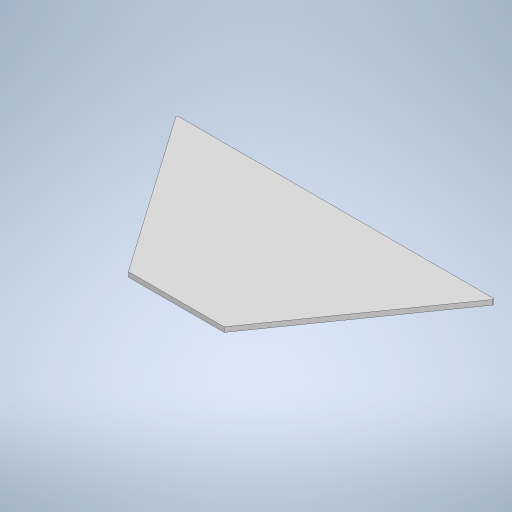
# Autodesk Inventor part: ДМС 304 торец лотка кормовой
Saved by Autodesk Inventor 2024.2 (Build 282272000, 272)
## iProperties
Created: 2024-05-13
Part Number: ДМС 304 торец лотка кормовой
Material: Generic
Document SubType Name: Sheet Metal
Designer: admin
Density: 1 g/cm^3
Sheet Metal Rule: Default
Appearance: Default
Author: admin
Autodesk Inventor part; units mm, degrees
ref_plane "YZ Plane" through (0, 0, 0) normal (1, 0, 0) x (0, 1, 0)
ref_plane "XZ Plane" through (0, 0, 0) normal (0, 1, 0) x (-1, 0, 0)
ref_plane "XY Plane" through (0, 0, 0) normal (0, 0, 1) x (1, 0, 0)
sketch "Sketch1" plane through (0, 0, 0) normal (0, 0, 1) x (1, 0, 0)
  line L0 (-100.0208, 100) -> (-30, 0)
  line L1 (-30, 0) -> (30, 0)
  line L2 (30, 0) -> (100.0208, 100)
  line L3 (100.0208, 100) -> (-100.0208, 100)
  point P0 (0, 0)
  point P1 (0, 0)
  point P2 (0, 100)
  dimension "d0" = 100
  dimension "d1" = 60
  dimension "d2" = 200.0415
  dimension "d4" = 125
  measures "d0" distance between parallel lines of L1 L3
  measures "d1" distance of L0.end L1.end
  measures "d2" distance of L2.end L0.start
  measures "d4" angle of L1 L0
extrude "Plate1" add sketch "Sketch1" along normal blind 3
chamfer "Chamfer1" distance 1 angle 45 2 edges at (-100.0208, 100, 1.5) (100.0208, 100, 1.5)
equation "\"d0\" = Лоток_высота"
equation "\"d1\" = Лоток_ширина_низ"
equation "\"d4\" = Лоток_угол"
equation "\"d3\" = Thickness"
equation "\"BendRadius\" = Thickness"
equation "\"BendReliefWidth\" = Thickness"
equation "\"BendReliefDepth\" = 0.5 * Thickness"
equation "\"CornerReliefSize\" = 4 * Thickness"
equation "\"MinimumRemnant\" = 2 * Thickness"
equation "\"TransitionRadius\" = BendRadius"
equation "\"JacobiRadiusSize\" = BendRadius"
equation "\"GapSize\" = Thickness"
equation "\"Лоток_высота\" = 100"
equation "\"Лоток_ширина_низ\" = 60"
equation "\"Лоток_угол\" = 125deg"
equation "\"Thickness\" = 3"
body "Solid1"
